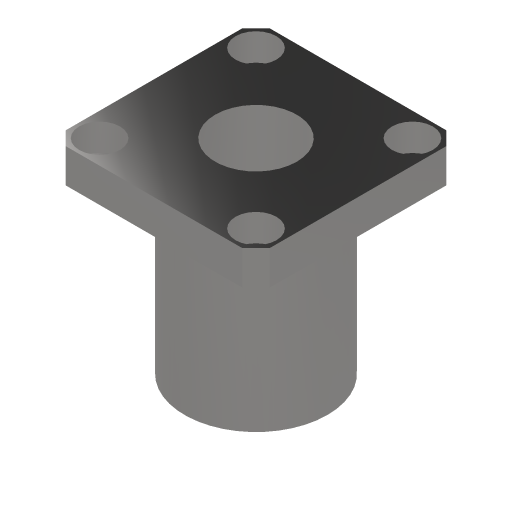
# Autodesk Inventor part: LM12UU
Saved by Autodesk Inventor 2023.2 (Build 272271000, 271)
## iProperties
Created: 2020-05-09
Part Number: LM12UU
Material: Stainless Steel
Document SubType Name: Modeling
Designer: Remo
Mass: 55.9832 g
Surface Area: 35.767 cm^2
Volume: 6.9979 cm^3
Density: 8 g/cm^3
Appearance: Semi-Polished
Author: Remo
Autodesk Inventor part; units mm, degrees
ref_plane "YZ Plane" through (0, 0, 0) normal (1, 0, 0) x (0, 1, 0)
ref_plane "XZ Plane" through (0, 0, 0) normal (0, 1, 0) x (-1, 0, 0)
ref_plane "XY Plane" through (0, 0, 0) normal (0, 0, 1) x (1, 0, 0)
sketch "Sketch1" plane through (0, 0, 0) normal (0, 0, 1) x (1, 0, 0)
  circle A0 centre (0, 0) radius 10.5
  circle A1 centre (0, 0) radius 6
  dimension "d0" = 12
  dimension "d1" = 21
  constraints: 2 centre point, 2 coincident
  measures "d0" diameter of A1
  measures "d1" diameter of A0
extrude "Extrusion1" add sketch "Sketch1" along normal blind 30
sketch "Sketch2" plane through (0, 0, 30) normal (0, 0, 1) x (1, 0, 0)
  circle A0 centre (0, 0) radius 6 projected
  circle A1 centre (0, 0) radius 10.5 projected
  line L0 (-15, -15) -> (15, -15)
  line L1 (15, -15) -> (15, 15)
  line L2 (15, 15) -> (-15, 15)
  line L3 (-15, 15) -> (-15, -15)
  line L4 (-15, -15) -> (15, 15) construction
  line L5 (15, -15) -> (-15, 15) construction
  dimension "d4" = 30
  constraints: 12 end point, 2 midpoint, 2 parallel, 2 perpendicular, 1 horizontal
  measures "d4" distance of L0.start L0.end
extrude "Extrusion2" add sketch "Sketch2" against normal blind 5 contours L3 L2 L1 L0
chamfer "Chamfer1" distance 2 angle 45 4 edges at (-15, 15, 27.5) (-15, -15, 27.5) (15, -15, 27.5) (15, 15, 27.5)
sketch "Sketch3" plane through (0, 0, 30) normal (0, 0, 1) x (1, 0, 0)
  point P0 (0, 0)
  point P1 (11.5, 11.5)
  point P2 (11.5, -11.5)
  point P3 (-11.5, -11.5)
  point P4 (-11.5, 11.5)
  dimension "d10" = 23
  dimension "d11" = 11.5
  dimension "d12" = 11.5
  dimension "d13" = 23
  constraints: 2 horizontal alignment, 2 vertical alignment
  measures "d10" distance of point (11.5, -11.5) point (11.5, 11.5)
  measures "d11" horizontal distance of point (11.5, 11.5) point (0, 0)
  measures "d12" horizontal distance of point (11.5, 11.5) point (0, 0)
  measures "d13" distance of point (11.5, 11.5) point (-11.5, 11.5)
hole "Hole1" at (11.5, 11.5, 30) at (11.5, -11.5, 30) at (-11.5, -11.5, 30) at (-11.5, 11.5, 30) direction (0, 0, -1) diameter 3 depth 8 tip angle 118 counterbore diameter 6 counterbore depth 4
equation "\"d11\" = 0.5 * d10"
equation "\"d12\" = d11"
equation "\"d13\" = d10"
body "Solid1"
